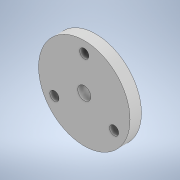
# Autodesk Inventor part: Disco da Valvula Inventor
Saved by Autodesk Inventor 2020 (Build 240168000, 168)
## iProperties
Created: 2022-04-28
Part Number: Disco da Valvula Inventor
Material: Genérico
Document SubType Name: Modeling
Designer: robofei
Density: 1 g/cm^3
Appearance: Padrão
Author: robofei
Autodesk Inventor part; units mm, degrees
ref_plane "YZ Plane" through (0, 0, 0) normal (1, 0, 0) x (0, 1, 0)
ref_plane "XZ Plane" through (0, 0, 0) normal (0, 1, 0) x (-1, 0, 0)
ref_plane "XY Plane" through (0, 0, 0) normal (0, 0, 1) x (1, 0, 0)
sketch "Esboço1" plane through (0, 0, 0) normal (0, 0, 1) x (1, 0, 0)
  circle A0 centre (0, 0) radius 14.34
  circle A1 centre (0, -0.3472) radius 100
  circle A2 centre (0, 75) radius 10
  circle A3 centre (-65.2526, -38.0208) radius 10
  circle A4 centre (65.2526, -38.0208) radius 10
  dimension "d0" = 200
  dimension "d1" = 20
  dimension "d2" = 75
  dimension "d5" = 360
  constraints: 5 centre point, 3 coincident, 8 other
  measures "d0" diameter of A1
  measures "d1" diameter of A2
  measures "d2" distance of point (0, 0) A2.centre
extrude "Extrusão1" add sketch "Esboço1" along normal blind 25
